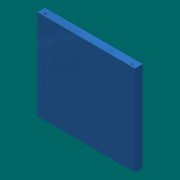
# Autodesk Inventor part: back
Saved by Autodesk Inventor 2016 (Build 200138000, 138)
## iProperties
Created: 2015-10-13
Part Number: back
Material: PC/ABS Plastic
Document SubType Name: Modeling
Designer: Sawaiz
Density: 0.357273 g/cm^3
Appearance: Cyan
Author: Sawaiz
Autodesk Inventor part; units mm, degrees
ref_plane "YZ Plane" through (0, 0, 0) normal (1, 0, 0) x (0, 1, 0)
ref_plane "XZ Plane" through (0, 0, 0) normal (0, 1, 0) x (-1, 0, 0)
ref_plane "XY Plane" through (0, 0, 0) normal (0, 0, 1) x (1, 0, 0)
sketch "Sketch1" plane through (0, 0, 0) normal (1, 0, 0) x (0, 1, 0)
  line L0 (-60.325, -55.5625) -> (60.325, -55.5625)
  line L1 (60.325, -55.5625) -> (60.325, 55.5625)
  line L2 (60.325, 55.5625) -> (-60.325, 55.5625)
  line L3 (-60.325, 55.5625) -> (-60.325, -55.5625)
  line L4 (-60.325, -55.5625) -> (60.325, 55.5625) construction
  line L5 (60.325, -55.5625) -> (-60.325, 55.5625) construction
  point P0 (0, 0)
  dimension "d0" = 120.65
  dimension "d1" = 111.125
  constraints: 12 end point, 2 midpoint, 2 parallel, 1 horizontal, 1 perpendicular
  measures "d0" distance of L2.end L1.end
  measures "d1" distance of L1.end L0.end
extrude "Extrusion1" add sketch "Sketch1" along normal blind 9.525
sketch "Sketch12" plane through (0, -60.325, 55.5625) normal (0, 0, 1) x (1, 0, 0)
  line L0 (0, 120.65) -> (9.525, 120.65) projected
  line L1 (0, 0) -> (9.525, 0) projected
  line L2 (0, 120.65) -> (0, 0) projected
  point P0 (0, 60.325)
  point P1 (6.35, 6.35)
  point P2 (6.35, 114.3)
  dimension "d131" = 6.35
  dimension "d139" = 6.35
  dimension "d140" = 6.35
  dimension "d141" = 6.35
  measures "d131" distance from line of L1 point (6.35, 6.35)
  measures "d139" distance from line of L2 point (6.35, 6.35)
  measures "d140" distance from line of L2 point (6.35, 114.3)
  measures "d141" distance from line of L0 point (6.35, 114.3)
hole "Hole6" at (6.35, -53.975, 55.5625) at (6.35, 53.975, 55.5625) direction (0, 0, -1) diameter 2.156 depth 8.865 tip angle 118 thread size "4-40 UNC" class "2B" standard "ANSI Unified Screw Threads"
equation "\"acrylicThickness\" = 9.525"
equation "\"height\" = 101.6"
equation "\"width\" = 101.6"
equation "\"depth\" = 203.2"
equation "\"mirrorAngle\" = 5deg"
equation "\"detectorWidth\" = 52"
equation "\"detectorHeight\" = 52"
equation "\"mirrorThickness\" = 3.175"
equation "\"fresnelThickness\" = 0.1"
equation "\"ior\" = 1.49"
equation "\"focalLength\" = 76.2"
equation "\"fresnelAngle\" = 90deg"
equation "\"centerThickness\" = 1.524"
equation "\"fresnelEffectiveDiameter\" = 76.2"
equation "\"mirrorSuppourtWidth\" = 38.1"
equation "\"backGrooveBit\" = 4.8006"
equation "\"sensorHolderHeight\" = 88.9"
equation "\"sensorHolderWidth\" = 88.9"
equation "\"sensorHolderSensorWidth\" = 53.975"
equation "\"sensorHolderSesnorHeight\" = 53.975"
equation "\"sensorHolderSensorHeight\" = 53.975"
equation "\"sensorHolderORingGroove\" = 3.175"
equation "\"sensorHolderORing\" = 3.175"
equation "\"sensorHolderFlushORingID\" = 304.8"
equation "\"sensorHolderFlushORing\" = 3.175"
equation "\"sensorHolderORingID\" = 203.2"
equation "\"oRingWidth\" = 1.5875"
equation "\"frontBackORingID\" = 419.1"
equation "\"topBottomHorizontalMirrorGroove\" = 12.7"
equation "\"backMirrorGroove\" = 6.35"
equation "\"mirrorGroove\" = 19.05"
equation "\"fresnelChamfer\" = 6.35"
equation "\"mirrorGrooveFillet\" = 6.35"
equation "\"mirrorGrooveDrill\" = 6.35"
equation "\"mirrorGrooveMill\" = 3.175"
equation "\"fresnelMirrorChamfer\" = 6.35"
equation "\"detectorOpeningWidth\" = 76.2"
equation "\"detectorOpeningHeight\" = 76.2"
equation "\"sensorHolderDepth\" = 19.05"
equation "\"internalAcrylicThicnkess\" = 6.35"
equation "\"frameAcrylicThickness\" = 9.525"
equation "\"aerogelHeight\" = 101.6"
equation "\"aerogelWidth\" = 101.6"
equation "\"internalAcrylicThickness\" = 6.35"
body "Solid1"
